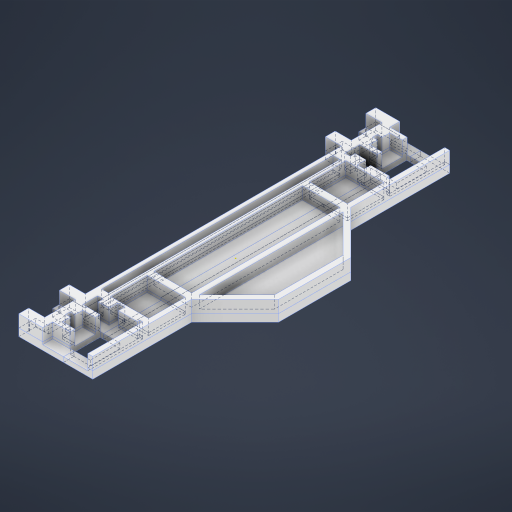
# Autodesk Inventor part: FlanecX_Aax
Saved by Autodesk Inventor 2024 (Build 280153000, 153)
## iProperties
Created: 2023-01-07
Part Number: FlanecX_Aax
Material: Aluminum 6061
Document SubType Name: Modeling
Designer: KirikDK
Density: 2.7 g/cm^3
Appearance: Aluminum - Flat
Mass: 6067.49 g
Surface Area: 4819.98 cm^2
Volume: 2247.22 cm^3
Author: KirikDK
Autodesk Inventor part; units mm, degrees
ref_plane "YZ Plane" through (0, 0, 0) normal (1, 0, 0) x (0, 1, 0)
ref_plane "XZ Plane" through (0, 0, 0) normal (0, 1, 0) x (-1, 0, 0)
ref_plane "XY Plane" through (0, 0, 0) normal (0, 0, 1) x (1, 0, 0)
sketch "Эскиз1" plane through (0, 0, 0) normal (0, 1, 0) x (-1, 0, 0)
  line L0 (45, 341) -> (-42, 341)
  line L1 (-42, 341) -> (-42, -381)
  line L2 (-42, -381) -> (45, -381)
  line L3 (45, -381) -> (45, 341)
  point P0 (0, 0)
  dimension "d0" = 87
  dimension "d1" = 722
  constraints: 8 end point, 2 parallel, 1 horizontal, 1 perpendicular
  measures "d0" distance of L0.start L0.end
  measures "d1" distance of L2.end L0.start
extrude "Выдавливание1" add sketch "Эскиз1" along normal blind 10
sketch "Эскиз2" plane through (0, 10, 0) normal (0, 1, 0) x (1, 0, 0)
  line L0 (26, -320) -> (-14, -320)
  line L1 (-14, -320) -> (-14, -260)
  line L2 (-14, -260) -> (26, -260)
  line L3 (26, -260) -> (26, -320)
  line L4 (-45, -341) -> (42, -341) projected
  line L5 (42, -341) -> (42, 381) projected
  line L6 (42, 381) -> (-45, 381) projected
  line L7 (-319, 20) -> (-306, 20)
  line L8 (26, 360) -> (-14, 360)
  line L9 (-14, 360) -> (-14, 300)
  line L10 (-14, 300) -> (26, 300)
  line L11 (26, 300) -> (26, 360)
  point P0 (0, 0)
  dimension "d4" = 21
  dimension "d5" = 16
  dimension "d6" = 60
  dimension "d7" = 40
  constraints: 18 end point, 4 symmetric about line, 2 horizontal, 2 parallel, 1 perpendicular
  measures "d4" distance between parallel lines of L4 L0
  measures "d5" distance between parallel lines of L5 L3
  measures "d6" distance of L2.end L0.start
  measures "d7" distance of L1.end L2.end
extrude "Выдавливание2" cut sketch "Эскиз2" against normal blind 10
sketch "Эскиз3" plane through (0, 10, 0) normal (0, 1, 0) x (1, 0, 0)
  line L0 (-45, 381) -> (-45, -341) projected
  line L1 (-45, -230) -> (-35, -230)
  line L2 (-35, -230) -> (-35, 270)
  line L3 (-35, 270) -> (-45, 270)
  line L4 (-45, 270) -> (-45, -230)
  line L5 (42, 381) -> (-45, 381) projected
  point P0 (0, 0)
  point P1 (-45, 270)
  dimension "d10" = 10
  dimension "d12" = 500
  dimension "d13" = 111
  constraints: 8 end point, 2 parallel, 1 horizontal, 1 perpendicular, 1 point on line
  measures "d10" distance between parallel lines of L0 L2
  measures "d12" distance of L1.end L2.end
  measures "d13" distance between parallel lines of L5 L3
extrude "Выдавливание3" add sketch "Эскиз3" along normal blind 25
sketch "Эскиз4" plane through (0, 0, 0) normal (0, -1, 0) x (1, 0, 0)
  line L0 (-45, -381) -> (-45, -270) projected
  line L1 (-45, -381) -> (-65, -381)
  line L2 (-65, -381) -> (-65, 341)
  line L3 (-65, 341) -> (-45, 341)
  line L4 (-45, 341) -> (-45, -381)
  line L5 (-45, 341) -> (42, 341) projected
  point P0 (0, 0)
  dimension "d16" = 722
  dimension "d17" = 0
  dimension "d20" = 20
  constraints: 8 end point, 2 parallel, 1 horizontal, 1 perpendicular, 1 point on line
  measures "d16" distance of L1.end L2.end
  measures "d17" distance between parallel lines of L3 L5
  measures "d20" distance of L1.start L1.end
extrude "Выдавливание4" add sketch "Эскиз4" against normal blind 35
sketch "Эскиз6" plane through (0, 0, 0) normal (0, -1, 0) x (1, 0, 0)
  line L0 (-45, 341) -> (42, 341) projected
  line L1 (42, 341) -> (52, 341)
  line L2 (52, 341) -> (52, -381)
  line L3 (52, -381) -> (42, -381)
  line L4 (42, -381) -> (42, 341)
  point P0 (0, 0)
  dimension "d22" = 10
  constraints: 8 end point, 2 parallel, 1 horizontal, 1 perpendicular
  measures "d22" distance of L2.end L3.end
extrude "Выдавливание5" add sketch "Эскиз6" against normal blind 40
sketch "Эскиз7" plane through (0, 10, 0) normal (0, 1, 0) x (1, 0, 0)
  line L0 (-35, -230) -> (-35, 270) projected
  line L1 (42, -341) -> (42, 381) projected
  line L2 (-35, 181) -> (42, 181)
  line L3 (42, 181) -> (42, -141)
  line L4 (42, -141) -> (-35, -141)
  line L5 (-35, -141) -> (-35, 181)
  line L6 (42, 381) -> (-45, 381) projected
  line L7 (-45, -341) -> (42, -341) projected
  line L8 (52, 181) -> (140, 181)
  line L9 (140, 181) -> (140, -141)
  line L10 (140, -141) -> (52, -141)
  line L11 (52, -141) -> (52, 181)
  point P0 (0, 0)
  point P1 (-35, -141)
  point P2 (42, 181)
  dimension "d25" = 200
  dimension "d26" = 200
  constraints: 16 end point, 4 parallel, 2 horizontal, 2 perpendicular, 2 point on line
  measures "d25" distance between parallel lines of L6 L2
  measures "d26" distance between parallel lines of L7 L4
extrude "Выдавливание6" add sketch "Эскиз7" along normal blind 5
sketch "Эскиз8" plane through (0, 15, 0) normal (0, 1, 0) x (1, 0, 0)
  line L0 (-18, 55) -> (24, 55)
  line L1 (24, 55) -> (24, -15)
  line L2 (24, -15) -> (-18, -15)
  line L3 (-18, -15) -> (-18, 55)
  line L4 (42, 381) -> (-45, 381) projected
  line L5 (19, -10) -> (19, 50)
  line L6 (19, 50) -> (-13, 50)
  line L7 (-13, 50) -> (-13, -10)
  line L8 (-13, -10) -> (19, -10)
  line L9 (1, 36) -> (-28.5, 36)
  line L10 (-28.5, 36) -> (-28.5, 4)
  line L11 (-28.5, 4) -> (1, 4)
  line L12 (1, 4) -> (1, 36)
  line L13 (-28.5, 36) -> (-18, 36)
  line L14 (-18, 36) -> (-18, 41)
  line L15 (-18, 41) -> (-28.5, 41)
  line L16 (-28.5, 41) -> (-28.5, 36)
  line L17 (-28.5, 4) -> (-18, 4)
  line L18 (-18, 4) -> (-18, -1)
  line L19 (-18, -1) -> (-28.5, -1)
  line L20 (-28.5, -1) -> (-28.5, 4)
  circle A0 centre (16, 50) radius 3
  circle A1 centre (-10, 50) radius 3
  circle A2 centre (-10, -10) radius 3
  circle A3 centre (16, -10) radius 3
  line L21 (92, 55) -> (134, 55)
  line L22 (134, 55) -> (134, -15)
  line L23 (134, -15) -> (92, -15)
  line L24 (92, -15) -> (92, 55)
  line L25 (129, -10) -> (129, 50)
  line L26 (129, 50) -> (97, 50)
  line L27 (97, 50) -> (97, -10)
  line L28 (97, -10) -> (129, -10)
  line L29 (111, 36) -> (81.5, 36)
  line L30 (81.5, 36) -> (81.5, 4)
  line L31 (81.5, 4) -> (111, 4)
  line L32 (111, 4) -> (111, 36)
  line L33 (81.5, 36) -> (92, 36)
  line L34 (92, 36) -> (92, 41)
  line L35 (92, 41) -> (81.5, 41)
  line L36 (81.5, 41) -> (81.5, 36)
  line L37 (81.5, 4) -> (92, 4)
  line L38 (92, 4) -> (92, -1)
  line L39 (92, -1) -> (81.5, -1)
  line L40 (81.5, -1) -> (81.5, 4)
  circle A4 centre (126, 50) radius 3
  circle A5 centre (100, 50) radius 3
  circle A6 centre (100, -10) radius 3
  circle A7 centre (126, -10) radius 3
  point P0 (0, 0)
  point P1 (-13, 36)
  point P2 (-7, 50)
  point P3 (13, 50)
  point P4 (13, -10)
  point P5 (-7, -10)
  point P6 (-13, 4)
  point P7 (97, 36)
  point P8 (103, 50)
  point P9 (123, 50)
  point P10 (123, -10)
  point P11 (103, -10)
  point P12 (97, 4)
  dimension "d29" = 42
  dimension "d30" = 70
  dimension "d31" = 326
  dimension "d32" = 5
  dimension "d33" = 10.5
  dimension "d47" = 5
  dimension "d48" = 5
  dimension "d49" = 19
  dimension "d50" = 19
  dimension "d61" = 42
  dimension "d62" = 70
  dimension "d63" = 5
  dimension "d64" = 10.5
  dimension "d65" = 5
  dimension "d66" = 5
  dimension "d67" = 19
  dimension "d68" = 19
  constraints: 80 end point, 20 parallel, 12 point on line, 10 perpendicular, 8 horizontal, 30 other
  measures "d29" distance of L0.start L0.end
  measures "d30" distance of L0.end L1.end
  measures "d31" distance between parallel lines of L0 L4
  measures "d32" distance between parallel lines of L1 L5
  measures "d33" distance between parallel lines of L3 L10
  measures "d47" distance between parallel lines of L9 L15
  measures "d48" distance between parallel lines of L19 L11
  measures "d49" distance between parallel lines of L2 L11
  measures "d50" distance between parallel lines of L0 L9
  measures "d61" distance of L21.start L21.end
  measures "d62" distance of L21.end L22.end
  measures "d63" distance between parallel lines of L22 L25
  measures "d64" distance between parallel lines of L24 L30
  measures "d65" distance between parallel lines of L29 L35
  measures "d66" distance between parallel lines of L39 L31
  measures "d67" distance between parallel lines of L23 L31
  measures "d68" distance between parallel lines of L21 L29
extrude "Выдавливание7" add sketch "Эскиз8" along normal blind 10 contours L0 L1 L2 L3 L11 L7 A2 L8 A3 L5 A0 L6 A1 L9 | L3 L9 L16 L15 | L3 L19 L20 L11 | L21 L22 L23 L24 L31 L27 A6 L28 A7 L25 A4 L26 A5 L29 | L24 L29 L36 L35 | L24 L39 L40 L31
sketch "Эскиз9" plane through (0, 15, 0) normal (0, 1, 0) x (1, 0, 0)
  line L0 (-8.75, 45.75) -> (14.75, 45.75)
  line L1 (14.75, 45.75) -> (14.75, -5.75)
  line L2 (14.75, -5.75) -> (-8.75, -5.75)
  line L3 (-8.75, -5.75) -> (-8.75, 45.75)
  line L4 (-28.5, 4) -> (-28.5, -1) projected
  line L5 (-28.5, -1) -> (-18, -1) projected
  line L6 (-18, -1) -> (-18, -15) projected
  line L7 (-18, -15) -> (24, -15) projected
  line L8 (24, -15) -> (24, 55) projected
  line L9 (24, 55) -> (-18, 55) projected
  line L10 (-18, 55) -> (-18, 41) projected
  line L11 (-18, 41) -> (-28.5, 41) projected
  line L12 (-28.5, 41) -> (-28.5, 36) projected
  line L13 (-28.5, 36) -> (-13, 36) projected
  line L14 (-13, 36) -> (-13, 50) projected
  arc A0 (-7, 50) -> (-13, 50) centre (-10, 50) ccw projected
  line L15 (-7, 50) -> (13, 50) projected
  arc A1 (19, 50) -> (13, 50) centre (16, 50) ccw projected
  line L16 (19, 50) -> (19, -10) projected
  arc A2 (13, -10) -> (19, -10) centre (16, -10) ccw projected
  line L17 (13, -10) -> (-7, -10) projected
  arc A3 (-13, -10) -> (-7, -10) centre (-10, -10) ccw projected
  line L18 (-13, -10) -> (-13, 4) projected
  line L19 (-13, 4) -> (-28.5, 4) projected
  circle A4 centre (-8.75, 45.75) radius 3.25
  circle A5 centre (14.75, 45.75) radius 3.25
  circle A6 centre (14.75, -5.75) radius 3.25
  circle A7 centre (-8.75, -5.75) radius 3.25
  circle A8 centre (-4.25, 20) radius 17
  line L20 (101.25, 45.75) -> (124.75, 45.75)
  line L21 (124.75, 45.75) -> (124.75, -5.75)
  line L22 (124.75, -5.75) -> (101.25, -5.75)
  line L23 (101.25, -5.75) -> (101.25, 45.75)
  circle A9 centre (101.25, 45.75) radius 3.25
  circle A10 centre (124.75, 45.75) radius 3.25
  circle A11 centre (124.75, -5.75) radius 3.25
  circle A12 centre (101.25, -5.75) radius 3.25
  circle A13 centre (105.75, 20) radius 17
  point P0 (0, 0)
  dimension "d36" = 4.25
  dimension "d37" = 4.25
  dimension "d38" = 4.25
  dimension "d39" = 4.25
  dimension "d40" = 19
  dimension "d41" = 34
  dimension "d69" = 19
  dimension "d70" = 34
  constraints: 16 end point, 10 centre point, 8 coincident, 4 parallel, 2 horizontal, 2 perpendicular
  measures "d36" distance between parallel lines of L15 L0
  measures "d37" distance between parallel lines of L17 L2
  measures "d38" distance between parallel lines of L16 L1
  measures "d39" distance between parallel lines of L18 L3
  measures "d40" distance from line of L1 A8.centre
  measures "d41" diameter of A8
  measures "d69" distance from line of L21 A13.centre
  measures "d70" diameter of A13
extrude "Выдавливание8" cut sketch "Эскиз9" against normal blind 20 contours L3 A4 L0 | L0 A4 L3 | A5 L1 L0 | L0 L1 A5 | A8 L3 | L3 A8 | A6 L2 L1 | L1 L2 A6 | A7 L2 L3 | L3 L2 A7 | L23 A9 L20 | L20 A9 L23 | A10 L21 L20 | L20 L21 A10 | A13 L23 | L23 A13 | A11 L22 L21 | L21 L22 A11 | A12 L22 L23 | L23 L22 A12
chamfer "Фаска1" [suppressed]
sketch "Эскиз10" plane through (-45, 10, -270) normal (1, 0, 0) x (0, 0, -1)
  line L0 (0, 25) -> (111, 25) projected
  line L1 (0, 0) -> (0, 25) projected
  line L2 (111, 0) -> (0, 0) projected
  line L3 (111, 0) -> (111, 25) projected
  line L4 (-611, 0) -> (-611, 25) projected
  line L5 (-500, 0) -> (-611, 0) projected
  line L6 (-500, 0) -> (-500, 25) projected
  line L7 (-611, 25) -> (-500, 25) projected
  line L8 (111, 0) -> (0, 0) projected
  line L9 (111, 0) -> (111, 25) projected
  line L10 (0, 25) -> (111, 25) projected
  line L11 (0, 0) -> (0, 25) projected
  line L12 (-500, 0) -> (-611, 0) projected
  line L13 (-500, 0) -> (-500, 25) projected
  line L14 (-611, 25) -> (-500, 25) projected
  line L15 (-611, 0) -> (-611, 25) projected
  point P0 (-270, -10)
extrude "Выдавливание9" cut sketch "Эскиз10" against normal blind 2
sketch "Эскиз12" plane through (0, 35, 0) normal (0, 1, 0) x (1, 0, 0)
  line L0 (-35, 270) -> (-45, 270) projected
  line L1 (-38, 270) -> (-16, 270)
  line L2 (-16, 270) -> (-16, 280)
  line L3 (-16, 280) -> (-38, 280)
  line L4 (-38, 280) -> (-38, 270)
  line L5 (35.9063, 275) -> (15.9063, 275)
  line L6 (15.9063, 275) -> (15.9063, 280)
  line L7 (15.9063, 280) -> (35.9063, 280)
  line L8 (35.9063, 280) -> (35.9063, 275)
  circle A0 centre (-4.25, 20) radius 17 projected
  line L9 (-4.25, 20) -> (0, 20)
  line L10 (-35, 269) -> (-35, 274.9994)
  line L11 (-35, 274.9994) -> (10.8519, 274.9994)
  line L12 (35.9063, 275) -> (-1.9378, 275)
  line L13 (-1.9378, 275) -> (-1.9378, 270)
  line L14 (-1.9378, 270) -> (35.9063, 270)
  line L15 (35.9063, 270) -> (35.9063, 275)
  line L16 (-35, -230) -> (-47, -230)
  line L17 (-38, -230) -> (-16, -230)
  line L18 (-16, -230) -> (-16, -240)
  line L19 (-16, -240) -> (-38, -240)
  line L20 (-38, -240) -> (-38, -230)
  line L21 (35.9063, -235) -> (15.9063, -235)
  line L22 (15.9063, -235) -> (15.9063, -240)
  line L23 (15.9063, -240) -> (35.9063, -240)
  line L24 (35.9063, -240) -> (35.9063, -235)
  line L25 (-35, -229) -> (-35, -234.9994)
  line L26 (-35, -234.9994) -> (10.8519, -234.9994)
  line L27 (35.9063, -235) -> (-1.9378, -235)
  line L28 (-1.9378, -235) -> (-1.9378, -230)
  line L29 (-1.9378, -230) -> (35.9063, -230)
  line L30 (35.9063, -230) -> (35.9063, -235)
  point P0 (0, 0)
  point P1 (-47, 270)
  point P2 (-16, -234.9994)
  point P3 (-35, -230)
  point P4 (-16, 274.9994)
  dimension "d56" = 10
  dimension "d57" = 20
  dimension "d58" = 5
  constraints: 60 end point, 16 symmetric about line, 6 parallel, 4 horizontal, 4 perpendicular, 4 point on line, 1 vertical
  measures "d56" distance of L1.end L2.end
  measures "d57" distance of L5.start L5.end
  measures "d58" distance of L5.end L6.end
extrude "Выдавливание11" add sketch "Эскиз12" against normal blind 25 contours L0 L4 L3 L2 L11 L10 | L15 L14 L13 L11 L12 L5 | L25 L26 L18 L19 L20 L16 | L21 L27 L26 L28 L29 L30
sketch "Sketch13" plane through (0, 15, 0) normal (0, 1, 0) x (1, 0, 0)
  point P0 (0, 0)
chamfer "Chamfer2" distance 88 angle 45 2 edges at (140, 12.5, -181) (140, 12.5, 141)
sketch "Sketch14" plane through (0, 0, 0) normal (0, -1, 0) x (1, 0, 0)
  line L0 (52, 141) -> (140, 53)
  line L1 (140, 53) -> (140, -93) projected
  line L2 (140, 53) -> (140, -93)
  line L3 (140, -93) -> (52, -181)
  line L4 (44.2218, 133.2218) -> (129, 48.4437)
  line L5 (129, 48.4437) -> (129, -88.4437)
  line L6 (129, -88.4437) -> (44.2218, -173.2218)
  line L7 (44.2218, -173.2218) -> (52, -181)
  line L8 (44.2218, 133.2218) -> (52, 141)
  line L9 (-35, -181) -> (42, -181) projected
  line L10 (42, -181) -> (-35, -181)
  line L11 (-35, -181) -> (-35, -170)
  line L12 (-35, -170) -> (42, -170)
  line L13 (42, -170) -> (42, -181)
  line L14 (42, 141) -> (-35, 141) projected
  line L15 (42, 141) -> (-35, 141)
  line L16 (-35, 141) -> (-35, 130)
  line L17 (-35, 130) -> (42, 130)
  line L18 (42, 130) -> (42, 141)
  point P0 (0, 0)
  dimension "d75" = 11
  dimension "d78" = 11
  dimension "d79" = 11
  constraints: 32 end point, 5 equal length, 5 perpendicular, 2 horizontal, 1 point on line, 2 other
  measures "d75" distance between parallel lines of L5 L1
  measures "d78" distance of L15.end L16.end
  measures "d79" distance of L10.end L11.end
extrude "Extrusion12" add sketch "Sketch14" against normal blind 40
sketch "Sketch15" plane through (-47, 10, -270) normal (1, 0, 0) x (0, 0, -1)
  line L0 (111, 25) -> (111, 0) projected
  line L1 (111, 25) -> (0, 25)
  line L2 (0, 25) -> (0, 0)
  line L3 (0, 0) -> (111, 0)
  line L4 (111, 0) -> (111, 25)
  line L5 (-500, 0) -> (-500, 25) projected
  line L6 (-611, 25) -> (-500, 25)
  line L7 (-500, 25) -> (-500, 0)
  line L8 (-500, 0) -> (-611, 0)
  line L9 (-611, 0) -> (-611, 25)
  point P0 (-270, -10)
  point P1 (111, 0)
  constraints: 16 end point, 4 parallel, 2 horizontal, 2 perpendicular
extrude "Extrusion13" cut sketch "Sketch15" against normal blind 2
sketch "Sketch16" plane through (0, 15, 0) normal (0, 1, 0) x (1, 0, 0)
  line L0 (-32, 62) -> (32, 62)
  line L1 (32, 62) -> (32, -29)
  line L2 (32, -29) -> (-32, -29)
  line L3 (-32, -29) -> (-32, 62)
  line L4 (129, -48.4437) -> (129, 88.4437) projected
  line L5 (75, 62) -> (129, 62)
  line L6 (129, 62) -> (129, -26)
  line L7 (129, -26) -> (75, -26)
  line L8 (75, -26) -> (75, 62)
  point P0 (0, 0)
  constraints: 16 end point, 4 parallel, 2 horizontal, 2 perpendicular, 2 point on line
extrude "Extrusion14" cut sketch "Sketch16" along normal blind 10
sketch "Sketch17" plane through (0, 15, 0) normal (0, 1, 0) x (1, 0, 0)
  line L0 (-24, 61) -> (29, 61)
  line L1 (29, 61) -> (29, -20)
  line L2 (29, -20) -> (-24, -20)
  line L3 (-24, -20) -> (-24, 61)
  line L4 (48.8801, 96.9843) -> (129.6537, 96.9843)
  line L5 (129.6537, 96.9843) -> (129.6537, -56.265)
  line L6 (129.6537, -56.265) -> (48.8801, -56.265)
  line L7 (48.8801, -56.265) -> (48.8801, 96.9843)
  line L8 (129.6537, -56.265) -> (48.6698, -137.249)
  line L9 (140, -53) -> (52, -141) projected
  line L10 (48.6698, -137.249) -> (48.6698, -56.265)
  line L11 (52, 165.4437) -> (52, -125.4437) projected
  line L12 (48.6698, -56.265) -> (129.6537, -56.265)
  line L13 (129.6537, 96.9843) -> (47, 177)
  line L14 (47, 177) -> (48.8801, 96.9843)
  line L15 (129.6537, 96.9843) -> (48.8801, 96.9843)
  point P0 (0, 0)
  constraints: 28 end point, 6 parallel, 3 perpendicular, 2 horizontal
extrude "Extrusion15" add sketch "Sketch17" against normal up to surface (15 mm away) contours L0 L1 L2 L3 | L4 L11 L6 L7 | L4 L5 L6 L11
sketch "Sketch18" plane through (0, 0, 0) normal (0, -1, 0) x (1, 0, 0)
  line L0 (-65, 341) -> (52, 341) projected
  line L1 (-65, -381) -> (52, -381) projected
  line L2 (24, -20) -> (-188, -20)
  line L3 (-65, 341) -> (-97.5, 341)
  line L4 (-97.5, 341) -> (-97.5, 320)
  line L5 (-97.5, 320) -> (-65, 320)
  line L6 (-65, 320) -> (-65, 341)
  line L7 (-65, 307) -> (-97.5, 307)
  line L8 (-97.5, 307) -> (-97.5, 273)
  line L9 (-97.5, 273) -> (-65, 273)
  line L10 (-65, 273) -> (-65, 307)
  line L11 (-97.5, 307) -> (-65, 307)
  line L12 (-65, 307) -> (-65, 320)
  line L13 (-65, 320) -> (-97.5, 320)
  line L14 (-97.5, 320) -> (-97.5, 307)
  line L15 (-97.5, 273) -> (-65, 273)
  line L16 (-65, 273) -> (-65, 260)
  line L17 (-65, 260) -> (-97.5, 260)
  line L18 (-97.5, 260) -> (-97.5, 273)
  line L19 (-72, 273) -> (-65, 273)
  line L20 (-65, 273) -> (-65, 307)
  line L21 (-65, 307) -> (-72, 307)
  line L22 (-72, 307) -> (-72, 273)
  line L23 (-97.5, 320) -> (-65, 341)
  line L24 (-97.5, 260) -> (-65, 238.9989)
  line L25 (-65, 341) -> (-65, -381) projected
  line L26 (-65, 260) -> (-65, 238.9989)
  line L27 (-65, -381) -> (-97.5, -381)
  line L28 (-97.5, -381) -> (-97.5, -360)
  line L29 (-97.5, -360) -> (-65, -360)
  line L30 (-65, -360) -> (-65, -381)
  line L31 (-65, -347) -> (-97.5, -347)
  line L32 (-97.5, -347) -> (-97.5, -313)
  line L33 (-97.5, -313) -> (-65, -313)
  line L34 (-65, -313) -> (-65, -347)
  line L35 (-97.5, -347) -> (-65, -347)
  line L36 (-65, -347) -> (-65, -360)
  line L37 (-65, -360) -> (-97.5, -360)
  line L38 (-97.5, -360) -> (-97.5, -347)
  line L39 (-97.5, -313) -> (-65, -313)
  line L40 (-65, -313) -> (-65, -300)
  line L41 (-65, -300) -> (-97.5, -300)
  line L42 (-97.5, -300) -> (-97.5, -313)
  line L43 (-72, -313) -> (-65, -313)
  line L44 (-65, -313) -> (-65, -347)
  line L45 (-65, -347) -> (-72, -347)
  line L46 (-72, -347) -> (-72, -313)
  line L47 (-97.5, -360) -> (-65, -381)
  line L48 (-97.5, -300) -> (-65, -278.9989)
  line L49 (-65, -300) -> (-65, -278.9989)
  point P0 (0, 0)
  dimension "d86" = 722
  dimension "d87" = 361
  dimension "d88" = 21
  dimension "d89" = 13
  dimension "d90" = 34
  dimension "d91" = 32.5
  dimension "d92" = 13
  dimension "d93" = 7
  dimension "d94" = 32.869
  dimension "d95" = 32.87
  constraints: 94 end point, 16 symmetric about line, 10 parallel, 6 horizontal, 6 point on line, 5 perpendicular, 1 vertical, 2 other
  measures "d86" distance between parallel lines of L0 L1
  measures "d87" distance between parallel lines of L1 L2
  measures "d88" distance between parallel lines of L5 L3
  measures "d89" distance between parallel lines of L7 L5
  measures "d90" distance between parallel lines of L9 L7
  measures "d91" distance between parallel lines of L6 L4
  measures "d92" distance between parallel lines of L17 L15
  measures "d93" distance between parallel lines of L20 L22
  measures "d94" angle of L23 L5
  measures "d95" angle of L17 L24
extrude "Extrusion16" add sketch "Sketch18" against normal blind 15 contours L6 L5 L23 | L12 L7 L14 L5 | L10 L9 L22 L7 | L16 L17 L18 L9 | L25 L24 L17 | L25 L41 L48 | L25 L33 L42 L41 | L25 L31 L46 L33 | L25 L29 L38 L31 | L25 L47 L29
sketch "Sketch19" plane through (0, 0, 0) normal (0, -1, 0) x (1, 0, 0)
  line L0 (-97.5, 260) -> (-97.5, 273) projected
  line L1 (-65, 238.9989) -> (-65, 341) projected
  line L2 (-97.5, 260) -> (-65, 260)
  line L3 (-65, 260) -> (-65, 242)
  line L4 (-65, 242) -> (-97.5, 242)
  line L5 (-97.5, 242) -> (-97.5, 260)
  line L6 (-97.5, 320) -> (-65, 320)
  line L7 (-65, 320) -> (-65, 338)
  line L8 (-65, 338) -> (-97.5, 338)
  line L9 (-97.5, 338) -> (-97.5, 320)
  line L10 (-97.5, -360) -> (-65, -381) projected
  line L11 (-97.5, -360) -> (-65, -360)
  line L12 (-65, -360) -> (-65, -378)
  line L13 (-65, -378) -> (-97.5, -378)
  line L14 (-97.5, -378) -> (-97.5, -360)
  line L15 (-65, -381) -> (-65, 341) projected
  line L16 (-97.5, -300) -> (-65, -300)
  line L17 (-65, -300) -> (-65, -282)
  line L18 (-65, -282) -> (-97.5, -282)
  line L19 (-97.5, -282) -> (-97.5, -300)
  line L20 (-65, 341) -> (-97.5, 320) projected
  line L21 (-97.5, 320) -> (-65, 320)
  line L22 (-65, 320) -> (-65, 321)
  line L23 (-65, 321) -> (-97.5, 321)
  line L24 (-97.5, 321) -> (-97.5, 320)
  line L25 (-97.5, 260) -> (-65, 260)
  line L26 (-65, 260) -> (-65, 259)
  line L27 (-65, 259) -> (-97.5, 259)
  line L28 (-97.5, 259) -> (-97.5, 260)
  line L29 (-97.5, -300) -> (-65, -278.9989) projected
  line L30 (-97.5, -300) -> (-65, -300)
  line L31 (-65, -300) -> (-65, -299)
  line L32 (-65, -299) -> (-97.5, -299)
  line L33 (-97.5, -299) -> (-97.5, -300)
  line L34 (-97.5, -360) -> (-65, -360)
  line L35 (-65, -360) -> (-65, -361)
  line L36 (-65, -361) -> (-97.5, -361)
  line L37 (-97.5, -361) -> (-97.5, -360)
  line L38 (-97.5, -299) -> (-65, -299)
  line L39 (-65, -299) -> (-65, -282)
  line L40 (-65, -282) -> (-97.5, -282)
  line L41 (-97.5, -282) -> (-97.5, -299)
  line L42 (-97.5, -361) -> (-65, -361)
  line L43 (-65, -361) -> (-65, -378)
  line L44 (-65, -378) -> (-97.5, -378)
  line L45 (-97.5, -378) -> (-97.5, -361)
  line L46 (-97.5, 259) -> (-65, 259)
  line L47 (-65, 259) -> (-65, 242)
  line L48 (-65, 242) -> (-97.5, 242)
  line L49 (-97.5, 242) -> (-97.5, 259)
  line L50 (-97.5, 321) -> (-65, 321)
  line L51 (-65, 321) -> (-65, 338)
  line L52 (-65, 338) -> (-97.5, 338)
  line L53 (-97.5, 338) -> (-97.5, 321)
  point P0 (0, 0)
  point P1 (-95.9525, -299)
  constraints: 96 end point, 24 parallel, 12 horizontal, 12 perpendicular, 4 point on line, 5 other
extrude "Extrusion18" add sketch "Sketch19" against normal up to surface (35 mm away) contours L4 L5 L27 L1 | L23 L20 L8 L1 | L23 L9 L8 L20 | L36 L12 L13 L10 | L10 L13 L14 L36 | L32 L29 L18 L15 | L32 L19 L18 L29
sketch "Sketch20" plane through (0, 0, 0) normal (0, -1, 0) x (1, 0, 0)
  line L0 (-97.5, 321) -> (-97.5, 338) projected
  line L1 (-65, 341) -> (52, 341) projected
  line L2 (-97.5, 338) -> (-65, 338)
  line L3 (-65, 338) -> (-65, 341)
  line L4 (-65, 341) -> (-97.5, 341)
  line L5 (-97.5, 341) -> (-97.5, 338)
  line L6 (-65, -378) -> (-97.5, -378) projected
  line L7 (-97.5, -378) -> (-65, -378)
  line L8 (-65, -378) -> (-65, -381)
  line L9 (-65, -381) -> (-97.5, -381)
  line L10 (-97.5, -381) -> (-97.5, -378)
  line L11 (-97.5, 242) -> (-65, 242)
  line L12 (-65, 242) -> (-65, 238.9989)
  line L13 (-65, 238.9989) -> (-97.5, 238.9989)
  line L14 (-97.5, 238.9989) -> (-97.5, 242)
  line L15 (-69.6443, -282) -> (-97.5, -282) projected
  line L16 (-65, -278.9989) -> (-69.6443, -282) projected
  line L17 (-97.5, -282) -> (-65, -282)
  line L18 (-65, -282) -> (-65, -278.9989)
  line L19 (-65, -278.9989) -> (-97.5, -278.9989)
  line L20 (-97.5, -278.9989) -> (-97.5, -282)
  point P0 (0, 0)
  constraints: 32 end point, 8 parallel, 4 horizontal, 4 perpendicular, 1 point on line
extrude "Extrusion19" add sketch "Sketch20" against normal up to surface (35 mm away)
sketch "Sketch21" plane through (0, 35, 0) normal (0, 1, 0) x (1, 0, 0)
  line L0 (-49, -341) -> (-49, -230) projected
  line L1 (-14, -320) -> (-14, -260) projected
  line L2 (-49, -321) -> (-14, -321)
  line L3 (-14, -321) -> (-14, -260)
  line L4 (-14, -260) -> (-49, -260)
  line L5 (-49, -260) -> (-49, -321)
  line L6 (42, -341) -> (-49, -341) projected
  line L7 (-38, -240) -> (-16, -240) projected
  line L8 (-49, -311) -> (-14, -311)
  line L9 (-14, -311) -> (-14, -270)
  line L10 (-14, -270) -> (-49, -270)
  line L11 (-49, -270) -> (-49, -311)
  line L12 (129, -48.4437) -> (129, 88.4437) projected
  line L13 (129, 88.4437) -> (52, 165.4437) projected
  line L14 (52, -125.4437) -> (52, 165.4437) projected
  line L15 (52, -125.4437) -> (129, -48.4437) projected
  line L16 (42, 381) -> (-49, 381) projected
  line L17 (82, 20) -> (116, 20)
  line L18 (-49, 381) -> (-49, 270)
  line L19 (-14, 360) -> (-14, 300)
  line L20 (-49, 361) -> (-14, 361)
  line L21 (-14, 361) -> (-14, 300)
  line L22 (-14, 300) -> (-49, 300)
  line L23 (-49, 300) -> (-49, 361)
  line L24 (42, 381) -> (-49, 381)
  line L25 (-38, 280) -> (-16, 280)
  line L26 (-49, 351) -> (-14, 351)
  line L27 (-14, 351) -> (-14, 310)
  line L28 (-14, 310) -> (-49, 310)
  line L29 (-49, 310) -> (-49, 351)
  line L30 (-49, -311) -> (-39, -311)
  line L31 (-39, -311) -> (-39, -270)
  line L32 (-39, -270) -> (-49, -270)
  line L33 (-49, -270) -> (-49, -311)
  line L34 (-49, 310) -> (-39, 310)
  line L35 (-39, 310) -> (-39, 351)
  line L36 (-39, 351) -> (-49, 351)
  line L37 (-49, 351) -> (-49, 310)
  line L38 (-49, -230) -> (-49, -341) projected
  line L39 (-49, -295) -> (-39, -295)
  line L40 (-39, -295) -> (-39, -286)
  line L41 (-39, -286) -> (-49, -286)
  line L42 (-49, -286) -> (-49, -295)
  line L43 (-49, 326) -> (-39, 326)
  line L44 (-39, 326) -> (-39, 335)
  line L45 (-39, 335) -> (-49, 335)
  line L46 (-49, 335) -> (-49, 326)
  line L47 (-1.9378, 270) -> (35.9063, 270) projected
  line L48 (42, 181) -> (42, 381) projected
  line L49 (-1.9378, 270) -> (42, 270)
  line L50 (42, 270) -> (42, 262)
  line L51 (42, 262) -> (-1.9378, 262)
  line L52 (-1.9378, 262) -> (-1.9378, 270)
  line L53 (-1.9378, -230) -> (42, -230)
  line L54 (42, -230) -> (42, -222)
  line L55 (42, -222) -> (-1.9378, -222)
  line L56 (-1.9378, -222) -> (-1.9378, -230)
  point P0 (0, 0)
  point P1 (-14, 351)
  point P2 (-14, -311)
  point P3 (-44, -311)
  dimension "d104" = 20
  dimension "d105" = 20
  dimension "d106" = 10
  dimension "d107" = 10
  dimension "d108" = 722
  dimension "d109" = 361
  dimension "d112" = 16
  dimension "d113" = 16
  dimension "d114" = 16
  dimension "d115" = 16
  constraints: 90 end point, 18 point on line, 16 parallel, 13 symmetric about line, 9 horizontal, 8 perpendicular, 1 midpoint
  measures "d104" distance between parallel lines of L6 L2
  measures "d105" distance between parallel lines of L7 L4
  measures "d106" distance between parallel lines of L4 L10
  measures "d107" distance between parallel lines of L2 L8
  measures "d108" distance between parallel lines of L16 L6
  measures "d109" distance between parallel lines of L17 L6
  measures "d112" distance between parallel lines of L36 L45
  measures "d113" distance between parallel lines of L34 L43
  measures "d114" distance between parallel lines of L32 L41
  measures "d115" distance from line of point (-44, -311) L39
extrude "Extrusion20" add sketch "Sketch21" against normal blind 30 contours L0 L8 L1 L3 L2 | L0 L39 L31 L8 | L0 L10 L31 L41 | L0 L4 L1 L10 | L20 L21 L19 L26 L18 | L26 L35 L45 L18 | L43 L35 L28 L18 | L28 L19 L22 L18 | L47 L49 L48 L51 L52 | L56 L55 L54 L53
sketch "Sketch23" plane through (0, 35, 0) normal (0, 1, 0) x (1, 0, 0)
  line L0 (-49, 270) -> (-49, 300) projected
  line L1 (-49, 300) -> (-14, 300) projected
  line L2 (-14, 300) -> (-14, 310) projected
  line L3 (-14, 310) -> (-39, 310) projected
  line L4 (-39, 310) -> (-39, 326) projected
  line L5 (-39, 326) -> (-49, 326) projected
  line L6 (-49, 326) -> (-49, 335) projected
  line L7 (-49, 335) -> (-39, 335) projected
  line L8 (-39, 335) -> (-39, 351) projected
  line L9 (-39, 351) -> (-14, 351) projected
  line L10 (-14, 351) -> (-14, 361) projected
  line L11 (-14, 361) -> (-49, 361) projected
  line L12 (-49, 361) -> (-49, 381) projected
  line L13 (-49, 381) -> (-97.5, 381) projected
  line L14 (-97.5, 381) -> (-97.5, 361) projected
  line L15 (-97.5, 361) -> (-65, 361) projected
  line L16 (-65, 361) -> (-65, 299) projected
  line L17 (-65, 299) -> (-97.5, 299) projected
  line L18 (-97.5, 299) -> (-97.5, 278.9989) projected
  line L19 (-97.5, 278.9989) -> (-65, 278.9989) projected
  line L20 (-65, 278.9989) -> (-65, -238.9989) projected
  line L21 (-65, -238.9989) -> (-97.5, -238.9989) projected
  line L22 (-97.5, -238.9989) -> (-97.5, -259) projected
  line L23 (-97.5, -259) -> (-65, -259) projected
  line L24 (-65, -259) -> (-65, -321) projected
  line L25 (-65, -321) -> (-97.5, -321) projected
  line L26 (-97.5, -321) -> (-97.5, -341) projected
  line L27 (-97.5, -341) -> (-49, -341) projected
  line L28 (-49, -341) -> (-49, -321) projected
  line L29 (-49, -321) -> (-14, -321) projected
  line L30 (-14, -321) -> (-14, -311) projected
  line L31 (-14, -311) -> (-39, -311) projected
  line L32 (-39, -311) -> (-39, -295) projected
  line L33 (-39, -295) -> (-49, -295) projected
  line L34 (-49, -295) -> (-49, -286) projected
  line L35 (-49, -286) -> (-39, -286) projected
  line L36 (-39, -286) -> (-39, -270) projected
  line L37 (-39, -270) -> (-14, -270) projected
  line L38 (-14, -270) -> (-14, -260) projected
  line L39 (-14, -260) -> (-49, -260) projected
  line L40 (-49, -260) -> (-49, -230) projected
  line L41 (-49, -230) -> (-38, -230) projected
  line L42 (-38, -230) -> (-38, -240) projected
  line L43 (-38, -240) -> (-16, -240) projected
  line L44 (-16, -240) -> (-16, -234.9994) projected
  line L45 (-16, -234.9994) -> (-35, -234.9994) projected
  line L46 (-35, -234.9994) -> (-35, -141) projected
  line L47 (-35, -141) -> (-35, -130) projected
  line L48 (-35, -130) -> (-35, 170) projected
  line L49 (-35, 170) -> (-35, 181) projected
  line L50 (-35, 181) -> (-35, 274.9994) projected
  line L51 (-35, 274.9994) -> (-16, 274.9994) projected
  line L52 (-16, 274.9994) -> (-16, 280) projected
  line L53 (-16, 280) -> (-38, 280) projected
  line L54 (-38, 280) -> (-38, 270) projected
  line L55 (-38, 270) -> (-49, 270) projected
  line L56 (-1.9378, -222) -> (-1.9378, -235) projected
  line L57 (-1.9378, -235) -> (35.9063, -235) projected
  line L58 (35.9063, -235) -> (35.9063, -230) projected
  line L59 (35.9063, -230) -> (42, -230) projected
  line L60 (42, -222) -> (42, -230) projected
  line L61 (42, -222) -> (-1.9378, -222) projected
  line L62 (35.9063, 275) -> (-1.9378, 275) projected
  line L63 (-1.9378, 275) -> (-1.9378, 262) projected
  line L64 (-1.9378, 262) -> (42, 262) projected
  line L65 (42, 270) -> (42, 262) projected
  line L66 (42, 270) -> (35.9063, 270) projected
  line L67 (35.9063, 270) -> (35.9063, 275) projected
  point P0 (0, 0)
extrude "Extrusion21" add sketch "Sketch23" along normal blind 5
sketch "Sketch24" plane through (0, 40, 0) normal (0, 1, 0) x (1, 0, 0)
  line L0 (-16, -234.9994) -> (-35, -234.9994) projected
  line L1 (-16, -234.9994) -> (-35, -234.9994)
  line L2 (-35, -234.9994) -> (-35, -218)
  line L3 (-35, -218) -> (-16, -218)
  line L4 (-16, -218) -> (-16, -234.9994)
  line L5 (42, -222) -> (-1.9378, -222) projected
  line L6 (-16, -218) -> (42, -218)
  line L7 (42, -218) -> (42, -222)
  line L8 (42, -222) -> (-16, -222)
  line L9 (-16, -222) -> (-16, -218)
  line L10 (-35, -141) -> (42, -141) projected
  line L11 (-35, -141) -> (42, -141)
  line L12 (42, -141) -> (42, -144)
  line L13 (42, -144) -> (-35, -144)
  line L14 (-35, -144) -> (-35, -141)
  line L15 (140, 20) -> (239, 20)
  line L16 (42, -130) -> (-35, -130) projected
  line L17 (42, -130) -> (41, -130)
  line L18 (41, -130) -> (41, 20)
  line L19 (41, 20) -> (42, 20)
  line L20 (42, 20) -> (42, -130)
  line L21 (121.1786, -56.265) -> (52, -125.4437) projected
  line L22 (127.9999, -49.4437) -> (140, -53)
  line L23 (140, 20) -> (116, 20)
  line L24 (140, -53) -> (140, 20)
  line L25 (127.9999, -49.4437) -> (127.9999, 20)
  line L26 (-16, 274.9994) -> (-35, 274.9994)
  line L27 (-16, 274.9994) -> (-35, 274.9994)
  line L28 (-35, 274.9994) -> (-35, 258)
  line L29 (-35, 258) -> (-16, 258)
  line L30 (-16, 258) -> (-16, 274.9994)
  line L31 (42, 262) -> (-1.9378, 262)
  line L32 (-16, 258) -> (42, 258)
  line L33 (42, 258) -> (42, 262)
  line L34 (42, 262) -> (-16, 262)
  line L35 (-16, 262) -> (-16, 258)
  line L36 (-35, 181) -> (42, 181)
  line L37 (-35, 181) -> (42, 181)
  line L38 (42, 181) -> (42, 184)
  line L39 (42, 184) -> (-35, 184)
  line L40 (-35, 184) -> (-35, 181)
  line L41 (42, 170) -> (-35, 170)
  line L42 (42, 170) -> (41, 170)
  line L43 (41, 170) -> (41, 20)
  line L44 (42, 20) -> (42, 170)
  line L45 (129, 88.4437) -> (52, 165.4437)
  line L46 (127.9999, 89.4437) -> (140, 93)
  line L47 (140, 93) -> (140, 20)
  line L48 (127.9999, 89.4437) -> (127.9999, 20)
  point P0 (0, 0)
  point P1 (129, -48.4437)
  point P2 (0, 40)
  constraints: 88 end point, 23 symmetric about line, 8 parallel, 6 horizontal, 5 perpendicular, 4 point on line, 1 midpoint, 1 vertical
extrude "Extrusion22" add sketch "Sketch24" against normal blind 30
sketch "Sketch28" plane through (0, 0, 0) normal (0, -1, 0) x (1, 0, 0)
  line L0 (126, -96) -> (49, -172)
  line L1 (49, -172) -> (47, 137)
  line L2 (47, 137) -> (131, 51.8947)
  line L3 (131, 51.8947) -> (126, -96)
  point P0 (0, 0)
  constraints: 8 end point, 1 perpendicular, 1 point on line
extrude "Extrusion26" add sketch "Sketch28" against normal up to surface (15 mm away)
sketch "Sketch30" plane through (52, 40, -381) normal (0, 0, -1) x (-1, 0, 0)
  line L0 (-93, -25) -> (154.5, -25)
  line L1 (154.5, -25) -> (154.5, -24.95)
  line L2 (154.5, -24.95) -> (-93, -24.95)
  line L3 (-93, -24.95) -> (-93, -25)
  line L4 (-88, 0) -> (-88, -40) projected
  line L5 (149.5, -40) -> (149.5, 0) projected
  point P0 (52, -40)
  point P1 (149.5, -20)
  dimension "d133" = 0.05
  dimension "d134" = 5
  dimension "d135" = 5
  constraints: 8 end point, 2 parallel, 1 horizontal, 1 midpoint, 1 perpendicular
  measures "d133" distance of L0.end L1.end
  measures "d134" distance between parallel lines of L4 L3
  measures "d135" distance from line of point (149.5, -20) L1
extrude "Extrusion27" cut sketch "Sketch30" against normal blind 1000
sketch "Sketch31" plane through (-49, 40, -381) normal (0, 0, -1) x (-1, 0, 0)
  line L0 (-42, -42) -> (-42.05, -42)
  line L1 (-42.05, -42) -> (-42.05, -24.9695)
  line L2 (-42.05, -24.9695) -> (-42, -24.9695)
  line L3 (-42, -24.9695) -> (-42, -42)
  line L4 (-47.0622, 0) -> (-33, 0) projected
  line L5 (48.5, -40) -> (-101, -40) projected
  point P0 (-49, -40)
  dimension "d138" = 0.05
  dimension "d140" = 2
  constraints: 8 end point, 2 parallel, 1 horizontal, 1 perpendicular
  measures "d138" distance of L0.start L0.end
  measures "d140" distance between parallel lines of L5 L0
extrude "Extrusion28" cut sketch "Sketch31" against normal blind 1000
sketch "Sketch32" plane through (0, 40, 0) normal (0, 1, 0) x (1, 0, 0)
  line L0 (-43, -214) -> (-57, -214)
  line L1 (-57, -214) -> (-57, 254)
  line L2 (-57, 254) -> (-43, 254)
  line L3 (-43, 254) -> (-43, -214)
  line L4 (-16, 262) -> (-16, 280) projected
  line L5 (-16, 280) -> (-38, 280) projected
  line L6 (-38, 280) -> (-38, 270) projected
  line L7 (-38, 270) -> (-49, 270) projected
  line L8 (-49, 270) -> (-49, 300) projected
  line L9 (-49, 300) -> (-14, 300) projected
  line L10 (-14, 300) -> (-14, 310) projected
  line L11 (-14, 310) -> (-39, 310) projected
  line L12 (-39, 310) -> (-39, 326) projected
  line L13 (-39, 326) -> (-49, 326) projected
  line L14 (-49, 326) -> (-49, 335) projected
  line L15 (-49, 335) -> (-39, 335) projected
  line L16 (-39, 335) -> (-39, 351) projected
  line L17 (-39, 351) -> (-14, 351) projected
  line L18 (-14, 351) -> (-14, 361) projected
  line L19 (-14, 361) -> (-49, 361) projected
  line L20 (-49, 361) -> (-49, 381) projected
  line L21 (-49, 381) -> (-97.5, 381) projected
  line L22 (-97.5, 381) -> (-97.5, 361) projected
  line L23 (-97.5, 361) -> (-65, 361) projected
  line L24 (-65, 361) -> (-65, 299) projected
  line L25 (-65, 299) -> (-97.5, 299) projected
  line L26 (-97.5, 299) -> (-97.5, 278.9989) projected
  line L27 (-97.5, 278.9989) -> (-65, 278.9989) projected
  line L28 (-65, 278.9989) -> (-65, -238.9989) projected
  line L29 (-65, -238.9989) -> (-97.5, -238.9989) projected
  line L30 (-97.5, -238.9989) -> (-97.5, -259) projected
  line L31 (-97.5, -259) -> (-65, -259) projected
  line L32 (-65, -259) -> (-65, -321) projected
  line L33 (-65, -321) -> (-97.5, -321) projected
  line L34 (-97.5, -321) -> (-97.5, -341) projected
  line L35 (-97.5, -341) -> (-49, -341) projected
  line L36 (-49, -341) -> (-49, -321) projected
  line L37 (-49, -321) -> (-14, -321) projected
  line L38 (-14, -321) -> (-14, -311) projected
  line L39 (-14, -311) -> (-39, -311) projected
  line L40 (-39, -311) -> (-39, -295) projected
  line L41 (-39, -295) -> (-49, -295) projected
  line L42 (-49, -295) -> (-49, -286) projected
  line L43 (-49, -286) -> (-39, -286) projected
  line L44 (-39, -286) -> (-39, -270) projected
  line L45 (-39, -270) -> (-14, -270) projected
  line L46 (-14, -270) -> (-14, -260) projected
  line L47 (-14, -260) -> (-49, -260) projected
  line L48 (-49, -260) -> (-49, -230) projected
  line L49 (-49, -230) -> (-38, -230) projected
  line L50 (-38, -230) -> (-38, -240) projected
  line L51 (-38, -240) -> (-16, -240) projected
  line L52 (-16, -240) -> (-16, -222) projected
  line L53 (-16, -222) -> (-1.9378, -222) projected
  line L54 (-1.9378, -222) -> (-1.9378, -235) projected
  line L55 (-1.9378, -235) -> (35.9063, -235) projected
  line L56 (35.9063, -235) -> (35.9063, -230) projected
  line L57 (35.9063, -230) -> (42, -230) projected
  line L58 (42, -230) -> (42, -341) projected
  line L59 (42, -341) -> (52, -341) projected
  line L60 (52, -341) -> (52, -141) projected
  line L61 (52, -141) -> (140, -53) projected
  line L62 (140, -53) -> (140, 93) projected
  line L63 (140, 93) -> (52, 181) projected
  line L64 (52, 181) -> (52, 381) projected
  line L65 (52, 381) -> (42, 381) projected
  line L66 (42, 381) -> (42, 270) projected
  line L67 (42, 270) -> (35.9063, 270) projected
  line L68 (35.9063, 270) -> (35.9063, 275) projected
  line L69 (35.9063, 275) -> (-1.9378, 275) projected
  line L70 (-1.9378, 275) -> (-1.9378, 262) projected
  line L71 (-1.9378, 262) -> (-16, 262) projected
  line L72 (-35, -218) -> (-35, -144) projected
  line L73 (-35, -144) -> (42, -144) projected
  line L74 (42, -144) -> (42, -218) projected
  line L75 (42, -218) -> (-35, -218) projected
  line L76 (-35, 258) -> (42, 258) projected
  line L77 (42, 258) -> (42, 184) projected
  line L78 (42, 184) -> (-35, 184) projected
  line L79 (-35, 184) -> (-35, 258) projected
  line L80 (127.9999, 89.4437) -> (127.9999, -49.4437) projected
  line L81 (127.9999, -49.4437) -> (52, -125.4437) projected
  line L82 (52, -125.4437) -> (52, 165.4437) projected
  line L83 (52, 165.4437) -> (127.9999, 89.4437) projected
  line L84 (-35, 170) -> (41, 170) projected
  line L85 (41, 170) -> (41, -130) projected
  line L86 (41, -130) -> (-35, -130) projected
  line L87 (-35, -130) -> (-35, 170) projected
  point P0 (0, 0)
  point P1 (-43.5, -230)
  dimension "d143" = 16
  dimension "d144" = 16
  dimension "d145" = 8
  dimension "d146" = 8
  constraints: 8 end point, 2 parallel, 1 horizontal, 1 midpoint, 1 perpendicular
  measures "d143" distance between parallel lines of L7 L2
  measures "d144" distance from line of point (-43.5, -230) L0
  measures "d145" distance between parallel lines of L28 L1
  measures "d146" distance between parallel lines of L3 L72
extrude "Extrusion29" cut sketch "Sketch32" against normal up to surface (30 mm away) contours L0 L1 L2 L3
